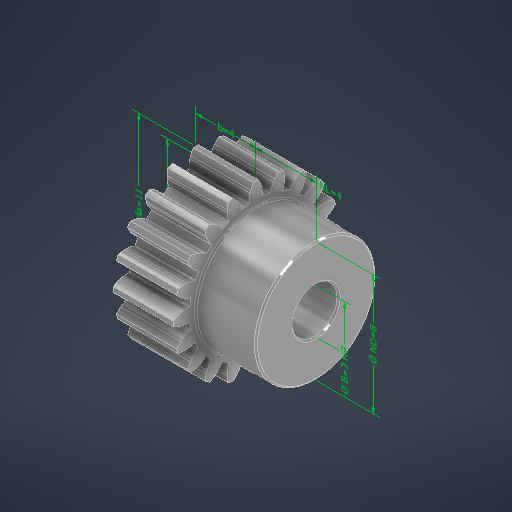
# Autodesk Inventor part: 21102000
Saved by Autodesk Inventor 2026.1 (Build 301233020, 233B)
## iProperties
Category: PARTsolutions
Company: MAEDLER
Created: 2025-12-15
Part Number: 21102000
Material: Generic
Catalog Web Link: www.3dfindit.com
Description: MAE-STZR-M0.5-MN-B4-ST-Spur Gears Made from Steel, with One-Sided Hub, Module 0.5, Tooth Width 4 mm
Vendor: MAEDLER
Document SubType Name: Modeling
Designer: psAdmin
Manufacturer: MAEDLER
Mass: 3 g
Surface Area: 5.64022 cm^2
Volume: 0.453362 cm^3
Density: 1 g/cm^3
Appearance: PSOLRGB-176-176-176
PSOL_IDENT_0: {$CADENAS_DATA/23d-libs/maedler/antriebselemente/stirnzahnraeder/stirnzahnraeder_stahl/modul_0_5_und
PSOL_IDENT_1: _0_7/stzr_m_0_5_zb4_st_mn.prj},173 {VTYP=3D},{NB=21102000},{LINA=21102000},{NN=MAE-STZR-M0.5-MN-B4-S
PSOL_IDENT_2: T},{DATE=31.10.2024 07:34:43},{GEOMDATE=31.10.2024 07:34:43},{VERSION=},{LINEID=100},{WBVAR=},{WBNUM
PSOL_IDENT_3: ERIC=}  {NB=21102000},{LINA=21102000},{KT=DUMMY},{ARTNR=21102000},{WEBSHOP=Produktdetails / Katalogs
PSOL_IDENT_4: eite / Montageanleitung},{MATK=Stahl},{MAT=Stahl 11SMn30+C (1.0715)},{M=0.5},{Z=20},{B=4},{DA=11.0},
PSOL_IDENT_5: {D=10.0},{NL=4},{ND=8},{BH7=3},{MD=2.2},{GEW=3.0},{CTN=84839089},{DIST=0.633},{GKD=9.39693},{FKD=8.8
PSOL_IDENT_6: 3300},{T0=1.57080},{UF=31.41593},{TLG=1.57080},{A=1.71010},{A3=0.57003},{PI=0.39270},{R2=0.04},{CNSD
PSOL_IDENT_7: WTEMPLATE=_dw/ansicht_right_front.dw}
NB: 21102000
NN: MAE-STZR-M0.5-MN-B4-ST
NT: Spur Gears Made from Steel, with One-Sided Hub, Module 0.5, Tooth Width 4 mm
NBSYN: $ARTNR.
LINA: 21102000
CATALOG: MÄDLER
ARTNR: 21102000
WEBSHOP: Product details / Catalogue page / Assembly instructions
MATK: Steel
MAT: Steel 11SMn30+C (1.0715)
M: 0.5
Z: 20
B: 4
DA: 11
D: 10
NL: 4
ND: 8
BH7: 3
MD: 2.2
GEW: 3
CTN: 84839089
SUPPLIER: MAEDLER
ARTICLENO: 21102000
BOMINFO: 21102000
CREATOR: CADENAS GmbH
Title: 21102000
Author: Cadenas PARTsolutions
Comments: Spur Gears Made from Steel, with One-Sided Hub, Module 0.5, Tooth Width 4 mm
Autodesk Inventor part; units mm, degrees
ref_plane "YZ Plane" through (0, 0, 0) normal (1, 0, 0) x (0, 1, 0)
ref_plane "XZ Plane" through (0, 0, 0) normal (0, 1, 0) x (-1, 0, 0)
ref_plane "XY Plane" through (0, 0, 0) normal (0, 0, 1) x (1, 0, 0)
sketch "Sketch_2" plane through (0, 0, 0) normal (0, 0, 1) x (1, 0, 0)
  line L0 (6, 0) -> (-2, 0)
  line L1 (-2, 5.5) -> (-2, 1.6061)
  line L2 (-2, 1.6061) -> (-1.8939, 1.5)
  line L3 (-1.8939, 1.5) -> (5.8939, 1.5)
  line L4 (5.8939, 1.5) -> (6, 1.6061)
  line L5 (6, 1.6061) -> (6, 3.8939)
  line L6 (6, 3.8939) -> (5.8939, 4)
  line L7 (5.8939, 4) -> (2.1, 4)
  arc A0 (2, 4.1) -> (2.1, 4) centre (2.1, 4.1) ccw
  line L8 (2, 4.1) -> (2, 5.5)
  line L9 (2, 5.5) -> (-2, 5.5)
  constraints: 20 end point, 2 point on circle, 1 centre point
revolve "Revolution1" add sketch "Sketch_2" angle 360 about axis through (6, 0, 0) along (1, 0, 0)
sketch "Sketch_4" plane through (0, 0, 0) normal (1, 0, 0) x (0, 0, -1)
  circle A0 centre (0, 0) radius 11
  arc A1 (-5.4974, 0.1681) -> (-5.4974, -0.1681) centre (0, 0) ccw
  arc A2 (-5.4974, -0.1681) -> (-5.136, -0.3426) centre (-4.4069, 1.6293) ccw
  arc A3 (-5.136, -0.3426) -> (-4.9846, -0.3923) centre (-4.5276, 1.2556) ccw
  arc A4 (-4.9846, -0.3923) -> (-4.4369, -0.4324) centre (-4.6166, 0.8731) ccw
  arc A5 (-4.3917, -0.4678) -> (-4.4369, -0.4324) centre (-4.4314, -0.472) ccw
  arc A6 (-4.3917, -0.4678) -> (-4.3213, -0.9122) centre (0, 0) ccw
  arc A7 (-4.3533, -0.9598) -> (-4.3213, -0.9122) centre (-4.3604, -0.9205) ccw
  arc A8 (-4.3533, -0.9598) -> (-4.8618, -1.1672) centre (-4.1209, -2.257) ccw
  arc A9 (-4.8618, -1.1672) -> (-4.9905, -1.2613) centre (-3.918, -2.5933) ccw
  arc A10 (-4.9905, -1.2613) -> (-5.2803, -1.5389) centre (-3.6877, -2.9114) ccw
  arc A11 (-5.2803, -1.5389) -> (-5.1764, -1.8587) centre (0, 0) ccw
  arc A12 (-5.1764, -1.8587) -> (-4.7787, -1.9129) centre (-4.6947, 0.1878) ccw
  arc A13 (-4.7787, -1.9129) -> (-4.6194, -1.9134) centre (-4.694, -0.2049) ccw
  arc A14 (-4.6194, -1.9134) -> (-4.0861, -1.7823) centre (-4.6605, -0.5962) ccw
  arc A15 (-4.0322, -1.802) -> (-4.0861, -1.7823) centre (-4.0687, -1.8183) ccw
  arc A16 (-4.0322, -1.802) -> (-3.8279, -2.2029) centre (0, 0) ccw
  arc A17 (-3.8437, -2.2581) -> (-3.8279, -2.2029) centre (-3.8626, -2.2229) ccw
  arc A18 (-3.8437, -2.2581) -> (-4.2632, -2.6125) centre (-3.2217, -3.42) ccw
  arc A19 (-4.2632, -2.6125) -> (-4.3565, -2.7417) centre (-2.9249, -3.6771) ccw
  arc A20 (-4.3565, -2.7417) -> (-4.5463, -3.0953) centre (-2.6076, -3.9085) ccw
  arc A21 (-4.5463, -3.0953) -> (-4.3487, -3.3673) centre (0, 0) ccw
  arc A22 (-4.3487, -3.3673) -> (-3.9537, -3.296) centre (-4.523, -1.2722) ccw
  arc A23 (-3.9537, -3.296) -> (-3.802, -3.2472) centre (-4.4009, -1.6454) ccw
  arc A24 (-3.802, -3.2472) -> (-3.3354, -2.9578) centre (-4.2481, -2.0072) ccw
  arc A25 (-3.278, -2.9598) -> (-3.3354, -2.9578) centre (-3.3077, -2.9866) ccw
  arc A26 (-3.278, -2.9598) -> (-2.9598, -3.278) centre (0, 0) ccw
  arc A27 (-2.9578, -3.3354) -> (-2.9598, -3.278) centre (-2.9866, -3.3077) ccw
  arc A28 (-2.9578, -3.3354) -> (-3.2472, -3.802) centre (-2.0072, -4.2481) ccw
  arc A29 (-3.2472, -3.802) -> (-3.296, -3.9537) centre (-1.6454, -4.4009) ccw
  arc A30 (-3.296, -3.9537) -> (-3.3673, -4.3487) centre (-1.2722, -4.523) ccw
  arc A31 (-3.3673, -4.3487) -> (-3.0953, -4.5463) centre (0, 0) ccw
  arc A32 (-3.0953, -4.5463) -> (-2.7417, -4.3565) centre (-3.9085, -2.6076) ccw
  arc A33 (-2.7417, -4.3565) -> (-2.6125, -4.2632) centre (-3.6771, -2.9249) ccw
  arc A34 (-2.6125, -4.2632) -> (-2.2581, -3.8437) centre (-3.42, -3.2217) ccw
  arc A35 (-2.2029, -3.8279) -> (-2.2581, -3.8437) centre (-2.2229, -3.8626) ccw
  arc A36 (-2.2029, -3.8279) -> (-1.802, -4.0322) centre (0, 0) ccw
  arc A37 (-1.7823, -4.0861) -> (-1.802, -4.0322) centre (-1.8183, -4.0687) ccw
  arc A38 (-1.7823, -4.0861) -> (-1.9134, -4.6194) centre (-0.5962, -4.6605) ccw
  arc A39 (-1.9134, -4.6194) -> (-1.9129, -4.7787) centre (-0.2049, -4.694) ccw
  arc A40 (-1.9129, -4.7787) -> (-1.8587, -5.1764) centre (0.1878, -4.6947) ccw
  arc A41 (-1.8587, -5.1764) -> (-1.5389, -5.2803) centre (0, 0) ccw
  arc A42 (-1.5389, -5.2803) -> (-1.2613, -4.9905) centre (-2.9114, -3.6877) ccw
  arc A43 (-1.2613, -4.9905) -> (-1.1672, -4.8618) centre (-2.5933, -3.918) ccw
  arc A44 (-1.1672, -4.8618) -> (-0.9598, -4.3533) centre (-2.257, -4.1209) ccw
  arc A45 (-0.9122, -4.3213) -> (-0.9598, -4.3533) centre (-0.9205, -4.3604) ccw
  arc A46 (-0.9122, -4.3213) -> (-0.4678, -4.3917) centre (0, 0) ccw
  arc A47 (-0.4324, -4.4369) -> (-0.4678, -4.3917) centre (-0.472, -4.4314) ccw
  arc A48 (-0.4324, -4.4369) -> (-0.3923, -4.9846) centre (0.8731, -4.6166) ccw
  arc A49 (-0.3923, -4.9846) -> (-0.3426, -5.136) centre (1.2556, -4.5276) ccw
  arc A50 (-0.3426, -5.136) -> (-0.1681, -5.4974) centre (1.6293, -4.4069) ccw
  arc A51 (-0.1681, -5.4974) -> (0.1681, -5.4974) centre (0, 0) ccw
  arc A52 (0.1681, -5.4974) -> (0.3426, -5.136) centre (-1.6293, -4.4069) ccw
  arc A53 (0.3426, -5.136) -> (0.3923, -4.9846) centre (-1.2556, -4.5276) ccw
  arc A54 (0.3923, -4.9846) -> (0.4324, -4.4369) centre (-0.8731, -4.6166) ccw
  arc A55 (0.4678, -4.3917) -> (0.4324, -4.4369) centre (0.472, -4.4314) ccw
  arc A56 (0.4678, -4.3917) -> (0.9122, -4.3213) centre (0, 0) ccw
  arc A57 (0.9598, -4.3533) -> (0.9122, -4.3213) centre (0.9205, -4.3604) ccw
  arc A58 (0.9598, -4.3533) -> (1.1672, -4.8618) centre (2.257, -4.1209) ccw
  arc A59 (1.1672, -4.8618) -> (1.2613, -4.9905) centre (2.5933, -3.918) ccw
  arc A60 (1.2613, -4.9905) -> (1.5389, -5.2803) centre (2.9114, -3.6877) ccw
  arc A61 (1.5389, -5.2803) -> (1.8587, -5.1764) centre (0, 0) ccw
  arc A62 (1.8587, -5.1764) -> (1.9129, -4.7787) centre (-0.1878, -4.6947) ccw
  arc A63 (1.9129, -4.7787) -> (1.9134, -4.6194) centre (0.2049, -4.694) ccw
  arc A64 (1.9134, -4.6194) -> (1.7823, -4.0861) centre (0.5962, -4.6605) ccw
  arc A65 (1.802, -4.0322) -> (1.7823, -4.0861) centre (1.8183, -4.0687) ccw
  arc A66 (1.802, -4.0322) -> (2.2029, -3.8279) centre (0, 0) ccw
  arc A67 (2.2581, -3.8437) -> (2.2029, -3.8279) centre (2.2229, -3.8626) ccw
  arc A68 (2.2581, -3.8437) -> (2.6125, -4.2632) centre (3.42, -3.2217) ccw
  arc A69 (2.6125, -4.2632) -> (2.7417, -4.3565) centre (3.6771, -2.9249) ccw
  arc A70 (2.7417, -4.3565) -> (3.0953, -4.5463) centre (3.9085, -2.6076) ccw
  arc A71 (3.0953, -4.5463) -> (3.3673, -4.3487) centre (0, 0) ccw
  arc A72 (3.3673, -4.3487) -> (3.296, -3.9537) centre (1.2722, -4.523) ccw
  arc A73 (3.296, -3.9537) -> (3.2472, -3.802) centre (1.6454, -4.4009) ccw
  arc A74 (3.2472, -3.802) -> (2.9578, -3.3354) centre (2.0072, -4.2481) ccw
  arc A75 (2.9598, -3.278) -> (2.9578, -3.3354) centre (2.9866, -3.3077) ccw
  arc A76 (2.9598, -3.278) -> (3.278, -2.9598) centre (0, 0) ccw
  arc A77 (3.3354, -2.9578) -> (3.278, -2.9598) centre (3.3077, -2.9866) ccw
  arc A78 (3.3354, -2.9578) -> (3.802, -3.2472) centre (4.2481, -2.0072) ccw
  arc A79 (3.802, -3.2472) -> (3.9537, -3.296) centre (4.4009, -1.6454) ccw
  arc A80 (3.9537, -3.296) -> (4.3487, -3.3673) centre (4.523, -1.2722) ccw
  arc A81 (4.3487, -3.3673) -> (4.5463, -3.0953) centre (0, 0) ccw
  arc A82 (4.5463, -3.0953) -> (4.3565, -2.7417) centre (2.6076, -3.9085) ccw
  arc A83 (4.3565, -2.7417) -> (4.2632, -2.6125) centre (2.9249, -3.6771) ccw
  arc A84 (4.2632, -2.6125) -> (3.8437, -2.2581) centre (3.2217, -3.42) ccw
  arc A85 (3.8279, -2.2029) -> (3.8437, -2.2581) centre (3.8626, -2.2229) ccw
  arc A86 (3.8279, -2.2029) -> (4.0322, -1.802) centre (0, 0) ccw
  arc A87 (4.0861, -1.7823) -> (4.0322, -1.802) centre (4.0687, -1.8183) ccw
  arc A88 (4.0861, -1.7823) -> (4.6194, -1.9134) centre (4.6605, -0.5962) ccw
  arc A89 (4.6194, -1.9134) -> (4.7787, -1.9129) centre (4.694, -0.2049) ccw
  arc A90 (4.7787, -1.9129) -> (5.1764, -1.8587) centre (4.6947, 0.1878) ccw
  arc A91 (5.1764, -1.8587) -> (5.2803, -1.5389) centre (0, 0) ccw
  arc A92 (5.2803, -1.5389) -> (4.9905, -1.2613) centre (3.6877, -2.9114) ccw
  arc A93 (4.9905, -1.2613) -> (4.8618, -1.1672) centre (3.918, -2.5933) ccw
  arc A94 (4.8618, -1.1672) -> (4.3533, -0.9598) centre (4.1209, -2.257) ccw
  arc A95 (4.3213, -0.9122) -> (4.3533, -0.9598) centre (4.3604, -0.9205) ccw
  arc A96 (4.3213, -0.9122) -> (4.3917, -0.4678) centre (0, 0) ccw
  arc A97 (4.4369, -0.4324) -> (4.3917, -0.4678) centre (4.4314, -0.472) ccw
  arc A98 (4.4369, -0.4324) -> (4.9846, -0.3923) centre (4.6166, 0.8731) ccw
  arc A99 (4.9846, -0.3923) -> (5.136, -0.3426) centre (4.5276, 1.2556) ccw
  arc A100 (5.136, -0.3426) -> (5.4974, -0.1681) centre (4.4069, 1.6293) ccw
  arc A101 (5.4974, -0.1681) -> (5.4974, 0.1681) centre (0, 0) ccw
  arc A102 (5.4974, 0.1681) -> (5.136, 0.3426) centre (4.4069, -1.6293) ccw
  arc A103 (5.136, 0.3426) -> (4.9846, 0.3923) centre (4.5276, -1.2556) ccw
  arc A104 (4.9846, 0.3923) -> (4.4369, 0.4324) centre (4.6166, -0.8731) ccw
  arc A105 (4.3917, 0.4678) -> (4.4369, 0.4324) centre (4.4314, 0.472) ccw
  arc A106 (4.3917, 0.4678) -> (4.3213, 0.9122) centre (0, 0) ccw
  arc A107 (4.3533, 0.9598) -> (4.3213, 0.9122) centre (4.3604, 0.9205) ccw
  arc A108 (4.3533, 0.9598) -> (4.8618, 1.1672) centre (4.1209, 2.257) ccw
  arc A109 (4.8618, 1.1672) -> (4.9905, 1.2613) centre (3.918, 2.5933) ccw
  arc A110 (4.9905, 1.2613) -> (5.2803, 1.5389) centre (3.6877, 2.9114) ccw
  arc A111 (5.2803, 1.5389) -> (5.1764, 1.8587) centre (0, 0) ccw
  arc A112 (5.1764, 1.8587) -> (4.7787, 1.9129) centre (4.6947, -0.1878) ccw
  arc A113 (4.7787, 1.9129) -> (4.6194, 1.9134) centre (4.694, 0.2049) ccw
  arc A114 (4.6194, 1.9134) -> (4.0861, 1.7823) centre (4.6605, 0.5962) ccw
  arc A115 (4.0322, 1.802) -> (4.0861, 1.7823) centre (4.0687, 1.8183) ccw
  arc A116 (4.0322, 1.802) -> (3.8279, 2.2029) centre (0, 0) ccw
  arc A117 (3.8437, 2.2581) -> (3.8279, 2.2029) centre (3.8626, 2.2229) ccw
  arc A118 (3.8437, 2.2581) -> (4.2632, 2.6125) centre (3.2217, 3.42) ccw
  arc A119 (4.2632, 2.6125) -> (4.3565, 2.7417) centre (2.9249, 3.6771) ccw
  arc A120 (4.3565, 2.7417) -> (4.5463, 3.0953) centre (2.6076, 3.9085) ccw
  arc A121 (4.5463, 3.0953) -> (4.3487, 3.3673) centre (0, 0) ccw
  arc A122 (4.3487, 3.3673) -> (3.9537, 3.296) centre (4.523, 1.2722) ccw
  arc A123 (3.9537, 3.296) -> (3.802, 3.2472) centre (4.4009, 1.6454) ccw
  arc A124 (3.802, 3.2472) -> (3.3354, 2.9578) centre (4.2481, 2.0072) ccw
  arc A125 (3.278, 2.9598) -> (3.3354, 2.9578) centre (3.3077, 2.9866) ccw
  arc A126 (3.278, 2.9598) -> (2.9598, 3.278) centre (0, 0) ccw
  arc A127 (2.9578, 3.3354) -> (2.9598, 3.278) centre (2.9866, 3.3077) ccw
  arc A128 (2.9578, 3.3354) -> (3.2472, 3.802) centre (2.0072, 4.2481) ccw
  arc A129 (3.2472, 3.802) -> (3.296, 3.9537) centre (1.6454, 4.4009) ccw
  arc A130 (3.296, 3.9537) -> (3.3673, 4.3487) centre (1.2722, 4.523) ccw
  arc A131 (3.3673, 4.3487) -> (3.0953, 4.5463) centre (0, 0) ccw
  arc A132 (3.0953, 4.5463) -> (2.7417, 4.3565) centre (3.9085, 2.6076) ccw
  arc A133 (2.7417, 4.3565) -> (2.6125, 4.2632) centre (3.6771, 2.9249) ccw
  arc A134 (2.6125, 4.2632) -> (2.2581, 3.8437) centre (3.42, 3.2217) ccw
  arc A135 (2.2029, 3.8279) -> (2.2581, 3.8437) centre (2.2229, 3.8626) ccw
  arc A136 (2.2029, 3.8279) -> (1.802, 4.0322) centre (0, 0) ccw
  arc A137 (1.7823, 4.0861) -> (1.802, 4.0322) centre (1.8183, 4.0687) ccw
  arc A138 (1.7823, 4.0861) -> (1.9134, 4.6194) centre (0.5962, 4.6605) ccw
  arc A139 (1.9134, 4.6194) -> (1.9129, 4.7787) centre (0.2049, 4.694) ccw
  arc A140 (1.9129, 4.7787) -> (1.8587, 5.1764) centre (-0.1878, 4.6947) ccw
  arc A141 (1.8587, 5.1764) -> (1.5389, 5.2803) centre (0, 0) ccw
  arc A142 (1.5389, 5.2803) -> (1.2613, 4.9905) centre (2.9114, 3.6877) ccw
  arc A143 (1.2613, 4.9905) -> (1.1672, 4.8618) centre (2.5933, 3.918) ccw
  arc A144 (1.1672, 4.8618) -> (0.9598, 4.3533) centre (2.257, 4.1209) ccw
  arc A145 (0.9122, 4.3213) -> (0.9598, 4.3533) centre (0.9205, 4.3604) ccw
  arc A146 (0.9122, 4.3213) -> (0.4678, 4.3917) centre (0, 0) ccw
  arc A147 (0.4324, 4.4369) -> (0.4678, 4.3917) centre (0.472, 4.4314) ccw
  arc A148 (0.4324, 4.4369) -> (0.3923, 4.9846) centre (-0.8731, 4.6166) ccw
  arc A149 (0.3923, 4.9846) -> (0.3426, 5.136) centre (-1.2556, 4.5276) ccw
  arc A150 (0.3426, 5.136) -> (0.1681, 5.4974) centre (-1.6293, 4.4069) ccw
  arc A151 (0.1681, 5.4974) -> (-0.1681, 5.4974) centre (0, 0) ccw
  arc A152 (-0.1681, 5.4974) -> (-0.3426, 5.136) centre (1.6293, 4.4069) ccw
  arc A153 (-0.3426, 5.136) -> (-0.3923, 4.9846) centre (1.2556, 4.5276) ccw
  arc A154 (-0.3923, 4.9846) -> (-0.4324, 4.4369) centre (0.8731, 4.6166) ccw
  arc A155 (-0.4678, 4.3917) -> (-0.4324, 4.4369) centre (-0.472, 4.4314) ccw
  arc A156 (-0.4678, 4.3917) -> (-0.9122, 4.3213) centre (0, 0) ccw
  arc A157 (-0.9598, 4.3533) -> (-0.9122, 4.3213) centre (-0.9205, 4.3604) ccw
  arc A158 (-0.9598, 4.3533) -> (-1.1672, 4.8618) centre (-2.257, 4.1209) ccw
  arc A159 (-1.1672, 4.8618) -> (-1.2613, 4.9905) centre (-2.5933, 3.918) ccw
  arc A160 (-1.2613, 4.9905) -> (-1.5389, 5.2803) centre (-2.9114, 3.6877) ccw
  arc A161 (-1.5389, 5.2803) -> (-1.8587, 5.1764) centre (0, 0) ccw
  arc A162 (-1.8587, 5.1764) -> (-1.9129, 4.7787) centre (0.1878, 4.6947) ccw
  arc A163 (-1.9129, 4.7787) -> (-1.9134, 4.6194) centre (-0.2049, 4.694) ccw
  arc A164 (-1.9134, 4.6194) -> (-1.7823, 4.0861) centre (-0.5962, 4.6605) ccw
  arc A165 (-1.802, 4.0322) -> (-1.7823, 4.0861) centre (-1.8183, 4.0687) ccw
  arc A166 (-1.802, 4.0322) -> (-2.2029, 3.8279) centre (0, 0) ccw
  arc A167 (-2.2581, 3.8437) -> (-2.2029, 3.8279) centre (-2.2229, 3.8626) ccw
  arc A168 (-2.2581, 3.8437) -> (-2.6125, 4.2632) centre (-3.42, 3.2217) ccw
  arc A169 (-2.6125, 4.2632) -> (-2.7417, 4.3565) centre (-3.6771, 2.9249) ccw
  arc A170 (-2.7417, 4.3565) -> (-3.0953, 4.5463) centre (-3.9085, 2.6076) ccw
  arc A171 (-3.0953, 4.5463) -> (-3.3673, 4.3487) centre (0, 0) ccw
  arc A172 (-3.3673, 4.3487) -> (-3.296, 3.9537) centre (-1.2722, 4.523) ccw
  arc A173 (-3.296, 3.9537) -> (-3.2472, 3.802) centre (-1.6454, 4.4009) ccw
  arc A174 (-3.2472, 3.802) -> (-2.9578, 3.3354) centre (-2.0072, 4.2481) ccw
  arc A175 (-2.9598, 3.278) -> (-2.9578, 3.3354) centre (-2.9866, 3.3077) ccw
  arc A176 (-2.9598, 3.278) -> (-3.278, 2.9598) centre (0, 0) ccw
  arc A177 (-3.3354, 2.9578) -> (-3.278, 2.9598) centre (-3.3077, 2.9866) ccw
  arc A178 (-3.3354, 2.9578) -> (-3.802, 3.2472) centre (-4.2481, 2.0072) ccw
  arc A179 (-3.802, 3.2472) -> (-3.9537, 3.296) centre (-4.4009, 1.6454) ccw
  arc A180 (-3.9537, 3.296) -> (-4.3487, 3.3673) centre (-4.523, 1.2722) ccw
  arc A181 (-4.3487, 3.3673) -> (-4.5463, 3.0953) centre (0, 0) ccw
  arc A182 (-4.5463, 3.0953) -> (-4.3565, 2.7417) centre (-2.6076, 3.9085) ccw
  arc A183 (-4.3565, 2.7417) -> (-4.2632, 2.6125) centre (-2.9249, 3.6771) ccw
  arc A184 (-4.2632, 2.6125) -> (-3.8437, 2.2581) centre (-3.2217, 3.42) ccw
  arc A185 (-3.8279, 2.2029) -> (-3.8437, 2.2581) centre (-3.8626, 2.2229) ccw
  arc A186 (-3.8279, 2.2029) -> (-4.0322, 1.802) centre (0, 0) ccw
  arc A187 (-4.0861, 1.7823) -> (-4.0322, 1.802) centre (-4.0687, 1.8183) ccw
  arc A188 (-4.0861, 1.7823) -> (-4.6194, 1.9134) centre (-4.6605, 0.5962) ccw
  arc A189 (-4.6194, 1.9134) -> (-4.7787, 1.9129) centre (-4.694, 0.2049) ccw
  arc A190 (-4.7787, 1.9129) -> (-5.1764, 1.8587) centre (-4.6947, -0.1878) ccw
  arc A191 (-5.1764, 1.8587) -> (-5.2803, 1.5389) centre (0, 0) ccw
  arc A192 (-5.2803, 1.5389) -> (-4.9905, 1.2613) centre (-3.6877, 2.9114) ccw
  arc A193 (-4.9905, 1.2613) -> (-4.8618, 1.1672) centre (-3.918, 2.5933) ccw
  arc A194 (-4.8618, 1.1672) -> (-4.3533, 0.9598) centre (-4.1209, 2.257) ccw
  arc A195 (-4.3213, 0.9122) -> (-4.3533, 0.9598) centre (-4.3604, 0.9205) ccw
  arc A196 (-4.3213, 0.9122) -> (-4.3917, 0.4678) centre (0, 0) ccw
  arc A197 (-4.4369, 0.4324) -> (-4.3917, 0.4678) centre (-4.4314, 0.472) ccw
  arc A198 (-4.4369, 0.4324) -> (-4.9846, 0.3923) centre (-4.6166, -0.8731) ccw
  arc A199 (-4.9846, 0.3923) -> (-5.136, 0.3426) centre (-4.5276, -1.2556) ccw
  arc A200 (-5.136, 0.3426) -> (-5.4974, 0.1681) centre (-4.4069, -1.6293) ccw
  constraints: 400 point on circle, 201 centre point
extrude "Extrusion1" cut sketch "Sketch_4" along normal mid plane 4
body "Solid1"
